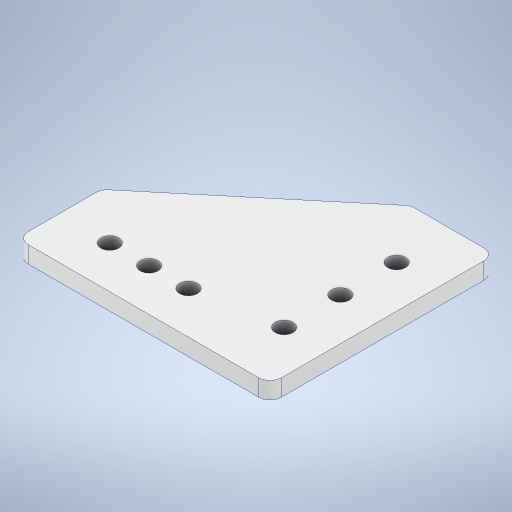
# Autodesk Inventor part: 射出_固定3
Saved by Autodesk Inventor 2023 (Build 270158000, 158)
## iProperties
Created: 2022-04-20
Part Number: 射出_固定3
Material: アルミニウム 6061
Document SubType Name: Modeling
Designer: yuta
Density: 2.7 g/cm^3
Appearance: アルミニウム - フラット
Author: yuta
Autodesk Inventor part; units mm, degrees
ref_plane "YZ Plane" through (0, 0, 0) normal (1, 0, 0) x (0, 1, 0)
ref_plane "XZ Plane" through (0, 0, 0) normal (0, 1, 0) x (-1, 0, 0)
ref_plane "XY Plane" through (0, 0, 0) normal (0, 0, 1) x (1, 0, 0)
sketch "スケッチ1" plane through (0, 0, 0) normal (0, 1, 0) x (-1, 0, 0)
  line L0 (0, 0) -> (45, 0)
  line L1 (45, 0) -> (45, -15)
  line L2 (0, -40) -> (0, 0)
  line L3 (45, 0) -> (45, -15)
  line L4 (45, 0) -> (60, 0) construction
  line L5 (0, -40) -> (15, -40)
  line L6 (0, -40) -> (15, -40) construction
  line L7 (15, -40) -> (45, -15)
  line L8 (15, -40) -> (0, -40)
  dimension "d2" = 15
  dimension "d3" = 90
  dimension "d4" = 15
  dimension "d5" = 0
  constraints: 18 end point, 3 horizontal, 2 collinear, 2 equal length, 2 parallel, 1 perpendicular
  measures "d2" distance of L0.end L1.end
  measures "d3" angle of L3 L4
  measures "d4" distance of L2.start L5.end
  measures "d5" distance between parallel lines of L5 L6
extrude "押し出し1" add sketch "スケッチ1" along normal blind 3
sketch "スケッチ2" plane through (0, 3, 0) normal (0, 1, 0) x (1, 0, 0)
  line L0 (-45, 0) -> (0, 0) projected
  line L1 (-45, 15) -> (-45, 0) projected
  line L2 (0, 0) -> (0, 40) projected
  line L3 (0, 40) -> (-15, 40) projected
  point P0 (-36, 7.5)
  point P1 (-7.5, 30)
  point P2 (-29, 7.5)
  point P3 (-22, 7.5)
  point P4 (-7.5, 20)
  point P5 (-7.5, 10)
  dimension "d8" = 7.5
  dimension "d9" = 9
  dimension "d10" = 7
  dimension "d11" = 7
  dimension "d12" = 7.5
  dimension "d13" = 7.5
  dimension "d14" = 7.5
  dimension "d15" = 10
  dimension "d16" = 10
  dimension "d17" = 10
  dimension "d18" = 7.5
  dimension "d19" = 7.5
  measures "d8" distance from line of L0 point (-36, 7.5)
  measures "d9" distance from line of L1 point (-36, 7.5)
  measures "d10" distance of point (-29, 7.5) point (-36, 7.5)
  measures "d11" distance of point (-22, 7.5) point (-29, 7.5)
  measures "d12" distance from line of L0 point (-29, 7.5)
  measures "d13" distance from line of L0 point (-22, 7.5)
  measures "d14" distance from line of L2 point (-7.5, 30)
  measures "d15" distance from line of L3 point (-7.5, 30)
  measures "d16" distance of point (-7.5, 20) point (-7.5, 30)
  measures "d17" distance of point (-7.5, 10) point (-7.5, 20)
  measures "d18" distance from line of L2 point (-7.5, 20)
  measures "d19" distance from line of L2 point (-7.5, 10)
hole "穴1" at (-36, 3, -7.5) at (-7.5, 3, -30) at (-29, 3, -7.5) at (-22, 3, -7.5) at (-7.5, 3, -20) at (-7.5, 3, -10) direction (0, -1, 0) diameter 3.2 end through all
fillet "フィレット1" radius 2 5 edges at (0, 1.5, -40) (0, 1.5, 0) (-45, 1.5, 0) (-45, 1.5, -15) (-15, 1.5, -40)
